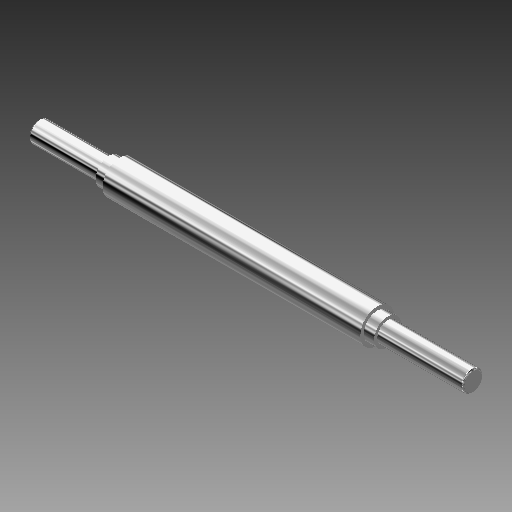
# Autodesk Inventor part: 401-04
Saved by Autodesk Inventor 2019 (Build 230136000, 136)
## iProperties
Company: Autodesk Inc.
Created: 2017-06-27
Part Number: 401-04
Material: Aluminum-6061
Document SubType Name: Modeling
Designer: Autodesk Inc.
Mass: 2.41256 g
Surface Area: 8.54618 cm^2
Volume: 0.89354 cm^3
Density: 2.7 g/cm^3
Appearance: Chrome - Polished
Author: Inventor
Autodesk Inventor part; units mm, degrees
ref_plane "YZ Plane" through (0, 0, 0) normal (1, 0, 0) x (0, 1, 0)
ref_plane "XZ Plane" through (0, 0, 0) normal (0, 1, 0) x (-1, 0, 0)
ref_plane "XY Plane" through (0, 0, 0) normal (0, 0, 1) x (1, 0, 0)
sketch "Sketch1" plane through (0, 0, 0) normal (0, 0, 1) x (1, 0, 0)
  line L0 (-18.55, 0) -> (18.55, 0)
  line L1 (18.55, 0) -> (18.55, 2.45)
  line L2 (18.55, 2.45) -> (-18.55, 2.45)
  line L3 (-18.55, 2.45) -> (-18.55, 0)
  line L4 (-18.55, 0) -> (-20.05, 0)
  line L5 (-20.05, 0) -> (-20.05, 1.95)
  line L6 (-20.05, 1.95) -> (-18.55, 1.95)
  line L7 (-18.55, 1.95) -> (-18.55, 0)
  line L8 (-20.05, 0) -> (-30.15, 0)
  line L9 (-30.15, 0) -> (-30.15, 1.5)
  line L10 (-30.15, 1.5) -> (-20.05, 1.5)
  line L11 (-20.05, 1.5) -> (-20.05, 0)
  line L12 (18.55, 0) -> (20.05, 0)
  line L13 (20.05, 0) -> (20.05, 1.95)
  line L14 (20.05, 1.95) -> (18.55, 1.95)
  line L15 (18.55, 1.95) -> (18.55, 0)
  line L16 (20.05, 0) -> (32.35, 0)
  line L17 (32.35, 0) -> (32.35, 1.5)
  line L18 (32.35, 1.5) -> (20.05, 1.5)
  line L19 (20.05, 1.5) -> (20.05, 0)
  point P0 (0, 0)
  point P1 (0, 0)
  dimension "d0" = 10.1
  dimension "d1" = 11.6
  dimension "d2" = 48.7
  dimension "d3" = 3
  dimension "d4" = 3.9
  dimension "d5" = 4.9
  dimension "d6" = 3
  dimension "d7" = 50.2
  dimension "d8" = 62.5
  constraints: 40 end point, 10 parallel, 5 horizontal, 5 perpendicular, 1 coincident, 1 collinear, 1 midpoint
  measures "d0" distance of L9.end L10.end
  measures "d1" distance between parallel lines of L3 L9
  measures "d2" distance between parallel lines of L1 L9
  measures "d3" diameter of L10 L8
  measures "d4" diameter of L6 L8
  measures "d5" diameter of L2 L8
  measures "d6" diameter of L18 L16
  measures "d7" distance between parallel lines of L19 L9
  measures "d8" distance between parallel lines of L9 L17
revolve "Revolution1" add sketch "Sketch1" angle 360 about axis through (-18.55, 0, 0) along (1, 0, 0)
fillet "Fillet1" radius 0.25 2 edges at (-30.15, -1.5, 0) (32.35, -1.5, 0)
body "Solid1"
